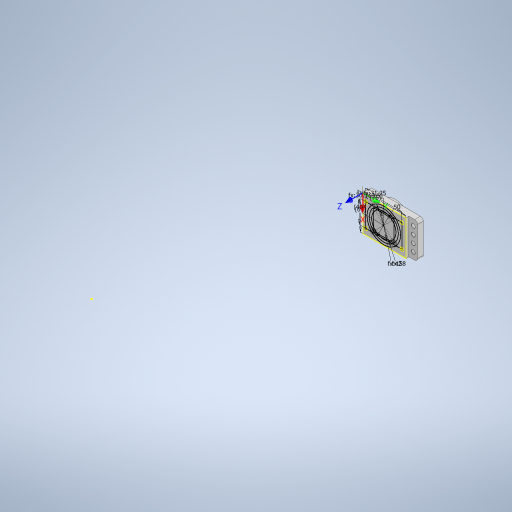
# Autodesk Inventor part: UR5 gripper mount
Saved by Autodesk Inventor 2024 (Build 280153000, 153)
## iProperties
Created: 2024-03-27
Part Number: UR5 gripper mount
Material: Generic
Document SubType Name: Modeling
Designer: jens1
Density: 1 g/cm^3
Appearance: Default
Author: jens1
## iProperties of the stored document UR5 gripper mount_3DPrint.ipt
Created: 2024-04-04
Part Number: UR5 gripper mount_3DPrint
Material: Generic
Document SubType Name: Modeling
Designer: jens1
Density: 1 g/cm^3
Appearance: Default
Author: jens1
Autodesk Inventor part; units mm, degrees
ref_plane "YZ Plane" through (0, 0, 0) normal (1, 0, 0) x (0, 1, 0)
ref_plane "XZ Plane" through (0, 0, 0) normal (0, 1, 0) x (-1, 0, 0)
ref_plane "XY Plane" through (0, 0, 0) normal (0, 0, 1) x (1, 0, 0)
sketch "Sketch1" plane through (0, 0, 0) normal (0, 0, 1) x (1, 0, 0)
  circle A0 centre (510.2334, 364.1488) radius 30.5 projected
  circle A1 centre (510.2334, 364.1488) radius 16.75 projected
  circle A2 centre (531.1627, 350.4752) radius 3.2 projected
  circle A3 centre (534.7013, 369.2793) radius 3.2 projected
  circle A4 centre (505.1029, 388.6167) radius 3.2 projected
  circle A5 centre (485.7655, 359.0183) radius 3.2 projected
  circle A6 centre (515.3639, 339.6809) radius 3.2 projected
  point P0 (0, 0)
extrude "Extrusion1" add sketch "Sketch1" along normal blind 10 contours A0 | A2
sketch "Sketch2" plane through (510.2334, 364.1488, 10) normal (0, 0, 1) x (1, 0, 0)
  line L0 (-40, -30.5) -> (40, -30.5)
  line L1 (40, -30.5) -> (40, 30.5)
  line L2 (40, 30.5) -> (-40, 30.5)
  line L3 (-40, 30.5) -> (-40, -30.5)
  line L4 (-40, -30.5) -> (40, 30.5) construction
  line L5 (40, -30.5) -> (-40, 30.5) construction
  circle A0 centre (0, 0) radius 30.5 projected
  circle A1 centre (0, 0) radius 30.5 projected
  circle A2 centre (0, 0) radius 16.75 projected
  circle A3 centre (24.4679, 5.1305) radius 3.2 projected
  circle A4 centre (-5.1305, 24.4679) radius 3.2 projected
  circle A5 centre (-24.4679, -5.1305) radius 3.2 projected
  circle A6 centre (5.1305, -24.4679) radius 3.2 projected
  point P0 (-510.2334, -364.1488)
  point P1 (0, 0)
  dimension "d2" = 80
  dimension "d3" = 0
  constraints: 12 end point, 2 midpoint, 2 parallel, 2 tangent, 1 horizontal, 1 perpendicular
  measures "d2" distance between parallel lines of L1 L3
  measures "d3" distance of A0.centre point (0, 0)
extrude "Extrusion2" add sketch "Sketch2" along normal blind 15
sketch "Sketch3" plane through (550.2334, 333.6488, 10) normal (1, 0, 0) x (0, 0, -1)
  line L0 (0, 0) -> (0, 61) projected
  line L1 (0, 61) -> (-15, 61) projected
  line L2 (-15, 0) -> (-15, 61) projected
  line L3 (0, 0) -> (-15, 0) projected
  line L4 (-15, 61) -> (-7.5, 61)
  line L5 (-7.5, 61) -> (-7.5, 0)
  line L6 (-7.5, 0) -> (-15, 0)
  line L7 (-15, 0) -> (-15, 61)
  line L8 (-15, 61) -> (-10, 61)
  line L9 (-10, 61) -> (-10, 0)
  line L10 (-10, 0) -> (-15, 0)
  line L11 (-15, 0) -> (-15, 61)
  point P0 (10, -333.6488)
  dimension "d34" = 5
  dimension "d35" = 15
  constraints: 16 end point, 4 parallel, 2 horizontal, 2 perpendicular, 1 midpoint, 1 point on line
  measures "d34" distance of L9.end L10.end
  measures "d35" distance between parallel lines of L2 L0
extrude "Extrusion3" add sketch "Sketch3" along normal blind 10 contours L3 L5 L1 L0 | L3 L9 L1 L5
fillet "Fillet1" radius 5 2 edges at (560.2334, 394.6488, 15) (560.2334, 333.6488, 15)
sketch "Sketch5" plane through (510.2334, 364.1488, 25) normal (0, 0, 1) x (1, 0, 0)
  point P0 (-510.2334, -364.1488)
sketch "Sketch6" plane through (550.2334, 333.6488, 10) normal (1, 0, 0) x (0, 0, -1)
  line L0 (-10, 0) -> (-15, 0) projected
  line L1 (-10, 61) -> (-15, 61) projected
  line L2 (-15, 0) -> (-15, 61) projected
  line L3 (-10, 0) -> (-10, 61) projected
  point P0 (10, -333.6488)
extrude "Extrusion5" cut sketch "Sketch6" against normal blind 5
sketch "Sketch9" plane through (510.2334, 364.1488, 10) normal (0, 0, -1) x (-1, 0, 0)
  line L0 (-50, 30.5) -> (-35, 30.5)
  line L1 (-35, 30.5) -> (-35, -30.5)
  line L2 (-35, -30.5) -> (-50, -30.5)
  line L3 (-50, -30.5) -> (-50, 30.5)
  line L4 (-50, -25.5) -> (-50, 25.5) projected
  line L5 (0, 30.5) -> (-45, 30.5) projected
  line L6 (0, -30.5) -> (-45, -30.5) projected
  line L7 (-50, 30.5) -> (-42.5, 30.5)
  line L8 (-42.5, 30.5) -> (-42.5, -30.5)
  line L9 (-42.5, -30.5) -> (-50, -30.5)
  line L10 (-50, -30.5) -> (-50, 30.5)
  point P0 (510.2334, -364.1488)
  point P1 (-50, 0)
  point P2 (-42.5, -19.5)
  point P3 (-42.5, -6.5)
  point P4 (-42.5, 6.5)
  point P5 (-42.5, 19.5)
  dimension "d49" = 15
  dimension "d50" = 13
  dimension "d51" = 13
  dimension "d52" = 13
  dimension "d53" = 61
  dimension "d54" = 11
  constraints: 16 end point, 6 point on line, 4 midpoint, 4 parallel, 2 horizontal, 2 perpendicular
  measures "d49" distance between parallel lines of L1 L3
  measures "d50" distance of point (-42.5, 19.5) point (-42.5, 6.5)
  measures "d51" distance of point (-42.5, -6.5) point (-42.5, 6.5)
  measures "d52" distance of point (-42.5, -19.5) point (-42.5, -6.5)
  measures "d53" distance of L2.end L0.start
  measures "d54" distance from line of L2 point (-42.5, -19.5)
hole "Hole4" at (552.7334, 383.6488, 10) at (552.7334, 370.6488, 10) at (552.7334, 357.6488, 10) at (552.7334, 344.6488, 10) direction (0, 0, 1) diameter 6 end through all
sketch "Sketch10" plane through (510.2334, 364.1488, 25) normal (0, 0, 1) x (1, 0, 0)
  point P0 (-510.2334, -364.1488)
sketch "Sketch11" plane through (510.2334, 364.1488, 25) normal (0, 0, 1) x (1, 0, 0)
  circle A0 centre (0, 0) radius 16.75 projected
  circle A1 centre (24.4679, 5.1305) radius 3.2 projected
  circle A2 centre (-5.1305, 24.4679) radius 3.2 projected
  circle A3 centre (-24.4679, -5.1305) radius 3.2 projected
  circle A4 centre (5.1305, -24.4679) radius 3.2 projected
  line L0 (35, -30.5) -> (35, 30.5) projected
  line L1 (35, 30.5) -> (-40, 30.5) projected
  line L2 (-40, 30.5) -> (-40, -30.5) projected
  line L3 (-40, -30.5) -> (35, -30.5) projected
  point P0 (-510.2334, -364.1488)
  point P1 (-35, 20)
  point P2 (-35, -20)
  point P3 (27.5, -20)
  point P4 (27.5, 20)
  dimension "d62" = 5
  dimension "d63" = 40
  dimension "d64" = 61
  dimension "d65" = 0
  dimension "d66" = 10.5
  dimension "d67" = 7.5
  dimension "d68" = 7.5
  dimension "d69" = 10.5
  dimension "d70" = 40
  measures "d62" distance from line of L2 point (-35, 20)
  measures "d63" distance of point (-35, -20) point (-35, 20)
  measures "d64" distance between parallel lines of L3 L1
  measures "d65" horizontal distance of point (-35, 20) point (-35, -20)
  measures "d66" distance from line of L3 point (-35, -20)
  measures "d67" distance from line of L0 point (27.5, -20)
  measures "d68" distance from line of L0 point (27.5, 20)
  measures "d69" distance from line of L1 point (27.5, 20)
  measures "d70" distance of point (27.5, -20) point (27.5, 20)
hole "Hole5" at (475.2334, 384.1488, 25) at (475.2334, 344.1488, 25) at (537.7334, 344.1488, 25) at (537.7334, 384.1488, 25) direction (0, 0, -1) diameter 5 end through all countersink diameter 6 countersink angle 90
sketch "Sketch12" plane through (510.2334, 364.1488, 25) normal (0, 0, 1) x (1, 0, 0)
  line L0 (17.6775, 17.6775) -> (-17.6775, 17.6775)
  line L1 (-17.6775, 17.6775) -> (-17.6775, -17.6775)
  line L2 (-17.6775, -17.6775) -> (17.6775, -17.6775)
  line L3 (17.6775, -17.6775) -> (17.6775, 17.6775)
  line L4 (17.6775, 17.6775) -> (-17.6775, -17.6775) construction
  line L5 (-17.6775, 17.6775) -> (17.6775, -17.6775) construction
  circle A0 centre (0, 0) radius 25
  circle A1 centre (0, 0) radius 16.75 projected
  point P0 (-510.2334, -364.1488)
  dimension "d78" = 35.355
  dimension "d79" = 35.355
  dimension "d80" = 50
  constraints: 12 end point, 5 coincident, 2 midpoint, 2 parallel, 1 centre point, 1 horizontal, 1 perpendicular
  measures "d78" distance of L2.end L1.end
  measures "d79" distance of L0.end L1.end
  measures "d80" diameter of A0
sketch "Sketch13" plane through (510.2334, 364.1488, 25) normal (0, 0, 1) x (1, 0, 0)
  circle A0 centre (27.5, 20) radius 3 projected
  circle A1 centre (27.5, -20) radius 3 projected
  circle A2 centre (-35, -20) radius 3 projected
  circle A3 centre (-35, 20) radius 3 projected
  circle A4 centre (0, 0) radius 16.75 projected
  circle A5 centre (24.4679, 5.1305) radius 3.2 projected
  circle A6 centre (-5.1305, 24.4679) radius 3.2 projected
  circle A7 centre (-24.4679, -5.1305) radius 3.2 projected
  circle A8 centre (5.1305, -24.4679) radius 3.2 projected
  line L0 (35, -30.5) -> (35, 30.5) projected
  line L1 (35, 30.5) -> (-40, 30.5) projected
  line L2 (-40, 30.5) -> (-40, -30.5) projected
  line L3 (-40, -30.5) -> (35, -30.5) projected
  point P0 (-510.2334, -364.1488)
extrude "Extrusion6" add sketch "Sketch13" against normal up to surface (25 mm away) contours A5 | A6 | A7 | A8
sketch "Sketch14" plane through (510.2334, 364.1488, 0) normal (0, 0, -1) x (-1, 0, 0)
  circle A0 centre (0, 0) radius 30.5 projected
  circle A1 centre (0, 0) radius 16.75 projected
  point P0 (510.2334, -364.1488)
extrude "Extrusion7" cut sketch "Sketch14" against normal up to surface (10 mm away)
sketch "Sketch15" plane through (510.2334, 364.1488, 10) normal (0, 0, -1) x (-1, 0, 0)
  circle A0 centre (0, 0) radius 16.75 projected
  point P0 (510.2334, -364.1488)
extrude "Extrusion8" add sketch "Sketch15" against normal up to surface (15 mm away)
sketch "Sketch16" plane through (510.2334, 364.1488, 25) normal (0, 0, 1) x (1, 0, 0)
  circle A0 centre (-3.75, 0) radius 25
  circle A1 centre (27.5, 20) radius 3 projected
  circle A2 centre (27.5, -20) radius 3 projected
  circle A3 centre (-35, -20) radius 3 projected
  circle A4 centre (-35, 20) radius 3 projected
  line L0 (35, -30.5) -> (35, 30.5) projected
  line L1 (35, 30.5) -> (-40, 30.5) projected
  line L2 (-40, 30.5) -> (-40, -30.5) projected
  line L3 (-40, -30.5) -> (35, -30.5) projected
  line L4 (-21.4277, -17.6777) -> (13.9277, -17.6777)
  line L5 (13.9277, -17.6777) -> (13.9277, 17.6777)
  line L6 (13.9277, 17.6777) -> (-21.4277, 17.6777)
  line L7 (-21.4277, 17.6777) -> (-21.4277, -17.6777)
  line L8 (-21.4277, -17.6777) -> (13.9277, 17.6777) construction
  line L9 (13.9277, -17.6777) -> (-21.4277, 17.6777) construction
  circle A5 centre (-3.75, 0) radius 29
  circle A6 centre (-3.75, 0) radius 21
  line L10 (27.5, 20) -> (-35, 20)
  line L11 (-35, 20) -> (-35, -20)
  line L12 (-35, -20) -> (27.5, -20)
  line L13 (27.5, -20) -> (27.5, 20)
  point P0 (-510.2334, -364.1488)
  dimension "d100" = 50
  dimension "d101" = 75
  dimension "d102" = 61
  dimension "d104" = 30.5
  dimension "d105" = 42
  dimension "d106" = 58
  dimension "d109" = 62.5
  dimension "d110" = 40
  dimension "d111" = 31.25
  constraints: 20 end point, 4 parallel, 3 perpendicular, 2 centre point, 2 coincident, 2 horizontal, 2 midpoint, 3 other
  measures "d101" distance of L0.end L1.end
  measures "d102" distance of L1.end L2.end
  measures "d104" distance from line of L1 point (-3.75, 0)
  measures "d105" diameter of A6
  measures "d106" diameter of A5
  measures "d109" distance of L10.start L10.end
  measures "d110" distance of L10.end L11.end
  measures "d111" distance from line of L11 point (-3.75, 0)
extrude "Extrusion9" add sketch "Sketch16" against normal blind 20 contours A0 L5 A6 | A0 L10 A5 L12 | L6 A6 L10 A0 | L5 A6 L6 | A0 L12 A6 L4 | L4 A6 L5 | L10 A6 A0 | A0 L10 A5 | L12 A5 A0 | A0 L12 A6 | L10 A6 L6 A0 | A0 L12 A5 L10 | A6 L7 L6 | A0 L4 A6 L12 | L4 L7 A6 | L7 A6 A0
hole "Hole7" at (488.8058, 381.8264, 25) at (488.8058, 346.4711, 25) at (524.1611, 346.4711, 25) at (524.1611, 381.8264, 25) direction (0, 0, -1) diameter 6.5 end through all counterbore diameter 11 counterbore depth 10
chamfer "Chamfer1" distance 0.5 angle 45 4 edges at (552.7334, 341.6488, 20) (552.7334, 354.6488, 20) (552.7334, 367.6488, 20) (552.7334, 380.6488, 20)
equation "\"d54\" = -1.5 * d52 + 0.5 * d53"
equation "\"d68\" = d67"
equation "\"d69\" = d66"
equation "\"d70\" = d63"
equation "\"d79\" = d78"
equation "\"d104\" = 0.5 * d102"
equation "\"d111\" = 0.5 * d109"
body "Solid1"
